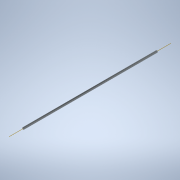
# Autodesk Inventor part: 细轴
Saved by Autodesk Inventor 2020 (Build 240168000, 168)
## iProperties
Created: 2012-04-11
Document SubType Name: Modeling
Designer: Autodesk Inc.
Density: 7.85 g/cm^3
Catalog Web Link: http://www.vexrobotics.com/shafts.html
Vendor: Innovation First, Inc.
Material: Steel
Mass: 23.9836 g
Surface Area: 37.5668 cm^2
Volume: 3.05523 cm^3
Appearance: 锌
Company: Autodesk Inc.
Category: Motion
Author: Autodesk Inc.
Autodesk Inventor part; units mm, degrees
ref_plane "YZ Plane" through (0, 0, 0) normal (1, 0, 0) x (0, 1, 0)
ref_plane "XZ Plane" through (0, 0, 0) normal (0, 1, 0) x (-1, 0, 0)
ref_plane "XY Plane" through (0, 0, 0) normal (0, 0, 1) x (1, 0, 0)
sketch "Sketch1" plane through (0, 0, 0) normal (0, 0, 1) x (1, 0, 0)
  line L0 (-1.5875, 0.3779) -> (-1.5875, -0.3779)
  arc A0 (-1.5875, -0.3779) -> (-0.3779, -1.5875) centre (0, 0) ccw
  line L1 (-0.3779, -1.5875) -> (0.3779, -1.5875)
  arc A1 (0.3779, -1.5875) -> (1.5875, -0.3779) centre (0, 0) ccw
  line L2 (1.5875, -0.3779) -> (1.5875, 0.3779)
  arc A2 (1.5875, 0.3779) -> (0.3779, 1.5875) centre (0, 0) ccw
  line L3 (0.3779, 1.5875) -> (-0.3779, 1.5875)
  arc A3 (-0.3779, 1.5875) -> (-1.5875, 0.3779) centre (0, 0) ccw
  arc A4 (-0.3779, 1.5875) -> (-1.5875, 0.3779) centre (0, 0) ccw
  line L4 (-1.3335, 1.5875) -> (-0.3779, 1.5875)
  spline S0 degree 3 poles (-1.3335, 1.5875) (-1.3642, 1.5875) (-1.3952, 1.5821) (-1.4569, 1.558) (-1.4873, 1.5388) (-1.5387, 1.4876) (-1.5579, 1.4569) (-1.582, 1.3955) (-1.5875, 1.3643) (-1.5875, 1.3335) knots 0 0 0 0 0.25 0.25 0.5 0.5 0.75 0.75 1 1 1 1
  line L5 (-1.5875, 0.3779) -> (-1.5875, 1.3335)
  line L6 (1.5875, 1.3335) -> (1.5875, 0.3779)
  spline S1 degree 3 poles (1.5875, 1.3335) (1.5875, 1.3642) (1.5821, 1.3952) (1.558, 1.4569) (1.5388, 1.4873) (1.4876, 1.5387) (1.4569, 1.5579) (1.3955, 1.582) (1.3643, 1.5875) (1.3335, 1.5875) knots 0 0 0 0 0.25 0.25 0.5 0.5 0.75 0.75 1 1 1 1
  line L7 (0.3779, 1.5875) -> (1.3335, 1.5875)
  arc A5 (1.5875, 0.3779) -> (0.3779, 1.5875) centre (0, 0) ccw
  spline S2 degree 3 poles (1.3335, -1.5875) (1.3642, -1.5875) (1.3952, -1.5821) (1.4569, -1.558) (1.4873, -1.5388) (1.5387, -1.4876) (1.5579, -1.4569) (1.582, -1.3955) (1.5875, -1.3643) (1.5875, -1.3335) knots 0 0 0 0 0.25 0.25 0.5 0.5 0.75 0.75 1 1 1 1
  line L8 (1.5875, -0.3779) -> (1.5875, -1.3335)
  arc A6 (0.3779, -1.5875) -> (1.5875, -0.3779) centre (0, 0) ccw
  line L9 (1.3335, -1.5875) -> (0.3779, -1.5875)
  spline S3 degree 3 poles (-1.5875, -1.3335) (-1.5875, -1.3642) (-1.5821, -1.3952) (-1.558, -1.4569) (-1.5388, -1.4873) (-1.4876, -1.5387) (-1.4569, -1.5579) (-1.3955, -1.582) (-1.3643, -1.5875) (-1.3335, -1.5875) knots 0 0 0 0 0.25 0.25 0.5 0.5 0.75 0.75 1 1 1 1
  line L10 (-0.3779, -1.5875) -> (-1.3335, -1.5875)
  arc A7 (-1.5875, -0.3779) -> (-0.3779, -1.5875) centre (0, 0) ccw
  line L11 (-1.5875, -1.3335) -> (-1.5875, -0.3779)
  constraints: 24 end point, 16 point on circle, 8 centre point, 8 other
extrude "Extrusion1" add sketch "Sketch1" against normal blind 304.8
ref_plane "Work Plane1" through (0, 0, 0) normal (0, 1, 0) x (0, 0, 1)
sketch "Sketch2" plane through (0, 0, 0) normal (0, 1, 0) x (0, 0, 1)
  spline S0 degree 3 poles (-0.1785, 2.0655) (-0.1352, 2.0163) (-0.1023, 1.9619) (-0.0534, 1.8515) (-0.0369, 1.7948) (-0.0026, 1.622) (0, 1.5057) (0, 1.3897) knots 0 0 0 0 0.25 0.25 0.5 0.5 1 1 1 1
  line L0 (0, 0) -> (0.3519, 0)
  line L1 (0.3519, 0) -> (0.3519, 2.1399)
  line L2 (0.3519, 2.1399) -> (-0.254, 2.1399)
  arc A0 (-0.1785, 2.0655) -> (-0.254, 2.1399) centre (-0.757, 1.5539) ccw
  line L3 (0, 0) -> (0, 1.3897)
  line L4 (-365.8304, 0) -> (61.3823, 0)
  point P0 (0, 0)
  constraints: 8 end point, 2 perpendicular, 2 point on circle, 1 centre point, 2 other
revolve "Revolution1" cut sketch "Sketch2" angle 360 about axis through (0, 0, 0) along (0, 0, 1)
ref_plane "工作平面3" through (0, 0, -304.8) normal (0, 0, 1) x (1, 0, 0)
split "分割1" plane through (0, 0, -304.8) removes the side toward (0, 0, -1)
equation "\"Length\" = 304.8"
equation "\"d4\" = -Length"
body "Solid1"
